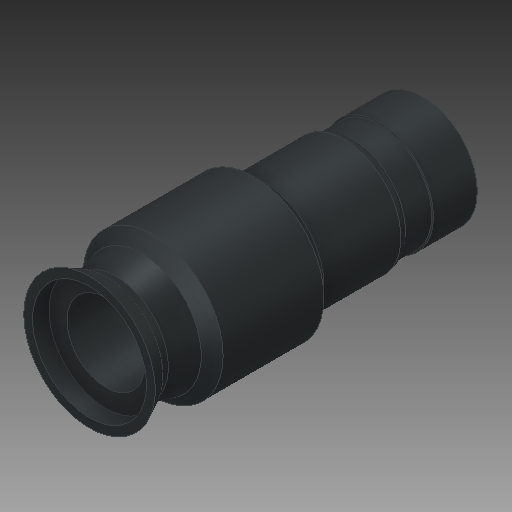
# Autodesk Inventor part: okular
Saved by Autodesk Inventor 2019.4 (Build 234330000, 330)
## iProperties
Created: 2019-06-01
Part Number: okular
Material: Iron, Cast
Document SubType Name: Modeling
Designer: Esterka
Density: 7.15 g/cm^3
Appearance: Iron Gray
Author: Esterka
Autodesk Inventor part; units mm, degrees
ref_plane "YZ Plane" through (0, 0, 0) normal (1, 0, 0) x (0, 1, 0)
ref_plane "XZ Plane" through (0, 0, 0) normal (0, 1, 0) x (-1, 0, 0)
ref_plane "XY Plane" through (0, 0, 0) normal (0, 0, 1) x (1, 0, 0)
sketch "Sketch1" plane through (0, 0, 0) normal (0, 0, 1) x (1, 0, 0)
  circle A0 centre (0, 0) radius 15.875
  dimension "d0" = 31.75
  constraints: 1 centre point, 1 coincident
  measures "d0" diameter of A0
extrude "Extrusion1" add sketch "Sketch1" along normal blind 20.32
sketch "Sketch2" plane through (0, 0, 20.32) normal (0, 0, 1) x (1, 0, 0)
  circle A0 centre (0, 0) radius 15.367
  circle A1 centre (0, 0) radius 16.7085
  dimension "d5" = 30.734
  constraints: 2 centre point, 2 coincident
  measures "d5" diameter of A0
extrude "Extrusion2" cut sketch "Sketch2" against normal blind 7.62
sketch "Sketch3" plane through (0, 0, 20.32) normal (0, 0, 1) x (1, 0, 0)
  circle A0 centre (0, 0) radius 16.51
  dimension "d6" = 33.02
  constraints: 1 centre point, 1 coincident
  measures "d6" diameter of A0
extrude "Extrusion3" add sketch "Sketch3" along normal blind 25.4
fillet "Fillet1" radius 3.175 1 edges at (-16.51, 0, 20.32)
sketch "Sketch4" plane through (0, 0, 45.72) normal (0, 0, 1) x (1, 0, 0)
  circle A0 centre (0, 0) radius 20.32
  dimension "d10" = 40.64
  constraints: 1 centre point, 1 coincident
  measures "d10" diameter of A0
extrude "Extrusion4" add sketch "Sketch4" along normal blind 35.56
chamfer "Chamfer1" distance 3.175 angle 45 2 edges at (-20.32, 0, 45.72) (-20.32, 0, 81.28)
sketch "Sketch5" plane through (0, 0, 0) normal (0, 1, 0) x (-1, 0, 0)
  point P0 (0, 0)
ref_plane "Work Plane1" through (0, 0, 88.9) normal (0, 0, 1) x (1, 0, 0)
sketch "Sketch6" plane through (0, 0, 88.9) normal (0, 0, 1) x (1, 0, 0)
  circle A0 centre (0, 0) radius 15.24
  dimension "d17" = 30.48
  constraints: 1 centre point, 1 coincident
  measures "d17" diameter of A0
loft "Loft1" add profiles "Sketch6" section 1 edges at (-17.145, 0, 81.28)
ref_plane "Work Plane2" through (0, 0, 96.52) normal (0, 0, 1) x (1, 0, 0)
sketch "Sketch7" plane through (0, 0, 96.52) normal (0, 0, 1) x (1, 0, 0)
  circle A0 centre (0, 0) radius 19.05
  dimension "d23" = 38.1
  constraints: 1 centre point, 1 coincident
  measures "d23" diameter of A0
loft "Loft2" add profiles "Sketch7" section 1 edges at (-15.24, 0, 88.9)
sketch "Sketch8" plane through (0, 0, 96.52) normal (0, 0, 1) x (1, 0, 0)
  circle A0 centre (0, 0) radius 16.51
  constraints: 1 centre point, 1 coincident
extrude "Extrusion5" cut sketch "Sketch8" against normal blind 4.7625
sketch "Sketch9" plane through (0, 0, 91.7575) normal (0, 0, 1) x (1, 0, 0)
  circle A0 centre (0, 0) radius 11.2811
  constraints: 1 centre point, 1 coincident
extrude "Extrusion6" cut sketch "Sketch9" against normal blind 120.65
body "Solid1"
